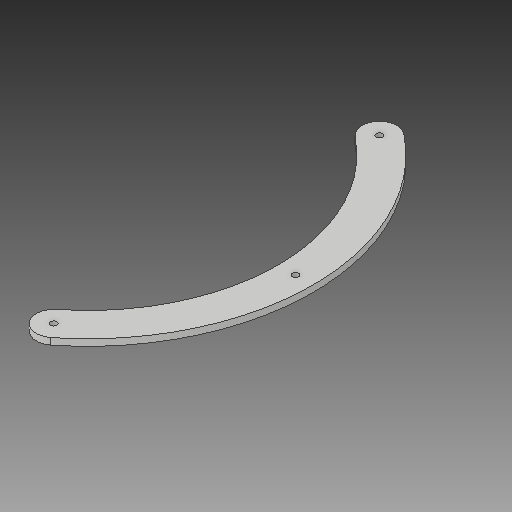
# Autodesk Inventor part: Arc
Saved by Autodesk Inventor 2018 (Build 220112000, 112)
## iProperties
Created: 2018-09-06
Part Number: Arc
Material: Generic
Document SubType Name: Modeling
Designer: matth
Density: 1 g/cm^3
Appearance: Default
Author: matth
Autodesk Inventor part; units mm, degrees
ref_plane "YZ Plane" through (0, 0, 0) normal (1, 0, 0) x (0, 1, 0)
ref_plane "XZ Plane" through (0, 0, 0) normal (0, 1, 0) x (-1, 0, 0)
ref_plane "XY Plane" through (0, 0, 0) normal (0, 0, 1) x (1, 0, 0)
sketch "Sketch1" plane through (0, 0, 0) normal (0, 1, 0) x (-1, 0, 0)
  arc A0 (-65, 70) -> (-65.0027, -69.9975) centre (0, 0) ccw
  line L0 (0, 0) -> (-65.0027, -69.9975) construction
  line L1 (0, 0) -> (-65, 70) construction
  circle A1 centre (-65, 70) radius 1.5
  circle A2 centre (-65.0027, -69.9975) radius 1.5
  arc A3 (-65, 70) -> (-65.0027, -69.9975) centre (0, 0) ccw construction
  arc A4 (-70.4436, 75.8623) -> (-70.4465, -75.8597) centre (0, 0) ccw
  arc A5 (-59.5564, 64.1377) -> (-59.5588, -64.1354) centre (0, 0) ccw
  arc A6 (-59.5564, 64.1377) -> (-70.4436, 75.8623) centre (-65, 70) ccw
  arc A7 (-70.4465, -75.8597) -> (-59.5588, -64.1354) centre (-65.0027, -69.9975) ccw
  dimension "d3" = 94.24
  dimension "d4" = 3
  dimension "d5" = 3
  dimension "d6" = 16
  constraints: 12 point on circle, 8 centre point, 5 tangent, 4 end point, 3 coincident
  measures "d3" angle of L1 L0
  measures "d4" diameter of A1
  measures "d5" diameter of A2
  measures "d6" diameter of A7
extrude "Extrusion1" add sketch "Sketch1" along normal blind 3
sketch "Sketch2" plane through (0, 3, 0) normal (0, 1, 0) x (1, 0, 0)
  circle A0 centre (65, -70) radius 1.5 projected
  circle A1 centre (0, 0) radius 95.5249
  line L0 (65, -70) -> (65, -75)
  line L1 (65, -75) -> (59.1608, -75)
  line L2 (65, 70) -> (65, 75)
  line L3 (65, 75) -> (59.1608, 75)
  arc A2 (59.1608, -75) -> (59.1608, 75) centre (0, 0) ccw construction
  arc A3 (64.1154, -81.2811) -> (64.1154, 81.2811) centre (0, 0) ccw
  arc A4 (54.2062, -68.7189) -> (54.2062, 68.7189) centre (0, 0) ccw
  arc A5 (54.2062, -68.7189) -> (64.1154, -81.2811) centre (59.1608, -75) ccw
  arc A6 (64.1154, 81.2811) -> (54.2062, 68.7189) centre (59.1608, 75) ccw
  circle A7 centre (65.0027, 69.9975) radius 1.5 projected
  circle A8 centre (65.0027, 69.9975) radius 1.5
  circle A9 centre (59.1608, 75) radius 1.5
  circle A10 centre (59.1608, -75) radius 1.5
  circle A11 centre (65, -70) radius 1.5
  dimension "d9" = 5
  dimension "d10" = 5
  dimension "d11" = 3
  dimension "d12" = 3
  dimension "d13" = 3
  constraints: 14 point on circle, 10 centre point, 8 end point, 5 coincident, 4 tangent, 2 perpendicular, 2 point on line, 1 concentric, 1 vertical
  measures "d9" distance of L0.start L0.end
  measures "d10" distance of L2.start L2.end
  measures "d11" diameter of A9
  measures "d12" diameter of A10
  measures "d13" diameter of A11
extrude "Extrusion2" add sketch "Sketch2" against normal blind 3 contours A0 A1 A7 L2 L3 A9 A6 A3 A5 A10 L1 L0 | A0 A1 A10 A5 A4 A6 A9 A7 | L0 L1 A10 A1 A0 | A1 A9 L3 L2 A7
sketch "Sketch3" plane through (0, 3, 0) normal (0, 1, 0) x (1, 0, 0)
  arc A0 (58.0606, -73.9805) -> (59.9988, -76.2441) centre (59.1608, -75) ccw projected
  circle A1 centre (59.1608, -75) radius 1.5
  arc A2 (65, -71.5) -> (63.8928, -71.012) centre (65, -70) ccw projected
  circle A3 centre (65, -70) radius 1.5
  arc A4 (63.8955, 71.0096) -> (65, 71.4975) centre (65.0027, 69.9975) ccw projected
  circle A5 centre (65.0027, 69.9975) radius 1.5
  arc A6 (60.002, 76.2419) -> (58.0631, 73.9777) centre (59.1608, 75) ccw projected
  circle A7 centre (59.1608, 75) radius 1.5
  point P0 (0, 0)
  constraints: 4 centre point, 4 coincident
extrude "Extrusion3" cut sketch "Sketch3" against normal blind 3
sketch "Sketch4" plane through (0, 3, 0) normal (0, 1, 0) x (1, 0, 0)
  circle A0 centre (65, -70) radius 1.5 projected
  circle A1 centre (65, -70) radius 1.5
  circle A2 centre (65.0027, 69.9975) radius 1.5 projected
  circle A3 centre (65.0027, 69.9975) radius 1.5
  point P0 (0, 0)
  constraints: 2 centre point, 2 coincident
extrude "Extrusion4" add sketch "Sketch4" against normal blind 3
sketch "Sketch5" plane through (0, 3, 0) normal (0, 1, 0) x (1, 0, 0)
  line L0 (0, 0) -> (95.525, 0)
  circle A0 centre (95.525, 0) radius 1.5
  dimension "d20" = 95.525
  dimension "d21" = 3
  constraints: 2 end point, 1 centre point, 1 coincident, 1 horizontal
  measures "d20" distance of L0.start L0.end
  measures "d21" diameter of A0
extrude "Extrusion5" cut sketch "Sketch5" against normal blind 3
body "Solid1"
